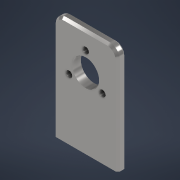
# Autodesk Inventor part: motorHolder_rotor
Saved by Autodesk Inventor 2021 (Build 250183000, 183)
## iProperties
Created: 2021-06-20
Part Number: motorHolder_rotor
Material: Steel, Mild
Document SubType Name: Modeling
Designer: Watchdog
Density: 7.85 g/cm^3
Appearance: Semi-Polished
Author: Watchdog
Autodesk Inventor part; units mm, degrees
ref_plane "YZ Plane" through (0, 0, 0) normal (1, 0, 0) x (0, 1, 0)
ref_plane "XZ Plane" through (0, 0, 0) normal (0, 1, 0) x (-1, 0, 0)
ref_plane "XY Plane" through (0, 0, 0) normal (0, 0, 1) x (1, 0, 0)
sketch "Sketch1" plane through (0, 0, 0) normal (0, 0, 1) x (1, 0, 0)
  line L0 (-30, 0) -> (30, 0)
  line L1 (30, 0) -> (30, 100)
  line L2 (30, 100) -> (-30, 100)
  line L3 (-30, 100) -> (-30, 0)
  point P0 (0, 0)
  dimension "d0" = 60
  dimension "d1" = 100
  dimension "d2" = 30
  constraints: 8 end point, 2 parallel, 1 horizontal, 1 midpoint, 1 perpendicular
  measures "d0" distance of L1.end L2.end
  measures "d1" distance of L0.end L1.end
  measures "d2" distance from line of point (0, 0) L3
extrude "Extrusion1" add sketch "Sketch1" along normal blind 8
fillet "Fillet1" radius 10 2 edges at (30, 100, 4) (-30, 100, 4)
sketch "Sketch2" plane through (0, 0, 8) normal (0, 0, 1) x (1, 0, 0)
  circle A0 centre (0, 66) radius 18
  line L0 (0, 66) -> (-15.5885, 57)
  line L1 (0, 66) -> (0, 84)
  line L2 (0, 66) -> (15.5885, 57)
  point P0 (0, 0)
  point P1 (0, 84)
  point P2 (-15.5885, 57)
  point P3 (15.5885, 57)
  dimension "d6" = 36
  dimension "d7" = 120
  dimension "d8" = 120
  dimension "d9" = 0
  dimension "d10" = 66
  constraints: 6 end point, 6 point on circle, 3 point on line, 1 centre point, 1 vertical
  measures "d6" diameter of A0
  measures "d7" angle of L1 L0
  measures "d8" angle of L2 L1
  measures "d9" horizontal distance of point (0, 0) L0.start
  measures "d10" distance of point (0, 0) L0.start
hole "Hole1" at (0, 84, 8) at (-15.5885, 57, 8) at (15.5885, 57, 8) direction (0, 0, -1) diameter 6 end through all
sketch "Sketch3" plane through (0, 0, 8) normal (0, 0, 1) x (1, 0, 0)
  circle A0 centre (0, 66) radius 12.5
  line L0 (-30, 0) -> (30, 0) projected
  point P0 (0, 0)
  dimension "d18" = 66
  dimension "d19" = 0
  dimension "d20" = 25
  constraints: 1 centre point
  measures "d18" distance from line of L0 A0.centre
  measures "d19" horizontal distance of point (0, 0) A0.centre
  measures "d20" diameter of A0
extrude "Extrusion2" cut sketch "Sketch3" against normal through all
chamfer "Chamfer1" distance 2 angle 45 10 edges at (0, 100, 8) (-27.0711, 97.0711, 8) (-30, 45, 8) (27.0711, 97.0711, 8) (30, 45, 8) (0, 100, 0) (-27.0711, 97.0711, 0) (-30, 45, 0) (27.0711, 97.0711, 0) (30, 45, 0)
equation "\"d2\" = 0.5 * d0"
equation "\"d10\" = centreHeight"
equation "\"d18\" = centreHeight"
equation "\"centreHeight\" = 66"
body "Solid1"
